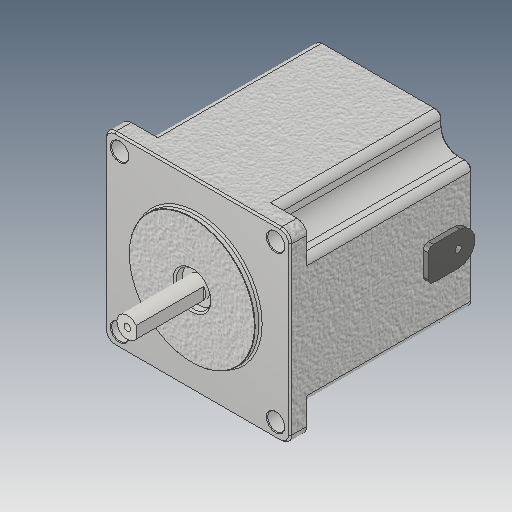
# Autodesk Inventor part: 23hs6403
Saved by Autodesk Inventor 2019 (Build 230136000, 136)
## iProperties
Created: 2018-10-14
Part Number: 23hs6403
Material: Generic
Document SubType Name: Modeling
Designer: LillaHunden
Density: 1 g/cm^3
Appearance: Default
Mass: 158.611 g
Surface Area: 187.385 cm^2
Volume: 158.611 cm^3
Author: LillaHunden
Autodesk Inventor part; units mm, degrees
ref_plane "YZ Plane" through (0, 0, 0) normal (1, 0, 0) x (0, 1, 0)
ref_plane "XZ Plane" through (0, 0, 0) normal (0, 1, 0) x (-1, 0, 0)
ref_plane "XY Plane" through (0, 0, 0) normal (0, 0, 1) x (1, 0, 0)
sketch "Sketch1" plane through (0, 0, 0) normal (0, 0, 1) x (1, 0, 0)
  line L0 (-28, -28) -> (28, -28)
  line L1 (28, -28) -> (28, 28)
  line L2 (28, 28) -> (-28, 28)
  line L3 (-28, 28) -> (-28, -28)
  line L4 (-28, -28) -> (28, 28) construction
  line L5 (28, -28) -> (-28, 28) construction
  point P0 (0, 0)
  dimension "d0" = 56
  dimension "d1" = 56
  constraints: 12 end point, 2 midpoint, 2 parallel, 1 horizontal, 1 perpendicular
  measures "d0" distance of L2.end L1.end
  measures "d1" distance of L1.end L0.end
extrude "Extrusion1" add sketch "Sketch1" along normal blind 55
sketch "Sketch2" plane through (0, 0, 55) normal (0, 0, 1) x (1, 0, 0)
  circle A0 centre (0, 0) radius 19
  dimension "d4" = 38
  constraints: 1 centre point, 1 coincident
  measures "d4" diameter of A0
extrude "Extrusion2" add sketch "Sketch2" along normal blind 1.7
fillet "Fillet1" radius 0.5 1 edges at (-19, 0, 55)
fillet "Fillet2" radius 0.1 1 edges at (-19, 0, 56.7)
sketch "Sketch3" plane through (0, 0, 56.7) normal (0, 0, 1) x (1, 0, 0)
  circle A0 centre (0, 0) radius 3.18
  dimension "d9" = 6.36
  constraints: 1 centre point, 1 coincident
  measures "d9" diameter of A0
extrude "Extrusion3" add sketch "Sketch3" along normal blind 19.5
sketch "Sketch4" plane through (0, 0, 56.7) normal (0, 0, 1) x (1, 0, 0)
  circle A0 centre (0, 0) radius 3.18 projected
  circle A1 centre (0, 0) radius 5.25
  dimension "d12" = 10.5
  constraints: 1 centre point, 1 coincident
  measures "d12" diameter of A1
extrude "Extrusion4" cut sketch "Sketch4" against normal blind 2.4
chamfer "Chamfer1" distance 0.5 angle 45 1 edges at (-5.25, 0, 56.7)
sketch "Sketch5" plane through (0, 0, 76.2) normal (0, 0, 1) x (1, 0, 0)
  circle A0 centre (0, 0) radius 1
  dimension "d18" = 2
  constraints: 1 centre point, 1 coincident
  measures "d18" diameter of A0
extrude "Extrusion5" cut sketch "Sketch5" against normal blind 2.4
draft "FaceDraft1" angle -20 pull direction (0, 0, -1) faces at (0.9871, -0.1604, 74.6) fixed edges at (-1, 0, 76.2)
sketch "Sketch6" plane through (0, 0, 55) normal (0, 0, 1) x (1, 0, 0)
  line L0 (-23.57, -23.57) -> (23.57, -23.57) construction
  line L1 (23.57, -23.57) -> (23.57, 23.57) construction
  line L2 (23.57, 23.57) -> (-23.57, 23.57) construction
  line L3 (-23.57, 23.57) -> (-23.57, -23.57) construction
  circle A0 centre (0, 0) radius 1 construction
  line L4 (-23.57, -23.57) -> (23.57, 23.57) construction
  line L5 (23.57, -23.57) -> (-23.57, 23.57) construction
  circle A1 centre (-23.57, 23.57) radius 2.6
  circle A2 centre (23.57, 23.57) radius 2.6
  circle A3 centre (23.57, -23.57) radius 2.6
  circle A4 centre (-23.57, -23.57) radius 2.6
  dimension "d22" = 47.14
  dimension "d23" = 47.14
  dimension "d24" = 5.2
  dimension "d25" = 5.2
  dimension "d26" = 5.2
  dimension "d27" = 5.2
  constraints: 12 end point, 4 centre point, 4 coincident, 2 midpoint, 2 parallel, 1 horizontal, 1 perpendicular
  measures "d22" distance of L2.end L1.end
  measures "d23" distance of L1.end L0.end
  measures "d24" diameter of A1
  measures "d25" diameter of A4
  measures "d26" diameter of A3
  measures "d27" diameter of A2
extrude "Extrusion6" cut sketch "Sketch6" against normal through all
chamfer "Chamfer2" distance 0.2 angle 45 4 edges at (-26.17, 23.57, 55) (20.97, 23.57, 55) (20.97, -23.57, 55) (-26.17, -23.57, 55)
sketch "Sketch7" plane through (0, 0, 0) normal (0, 0, -1) x (-1, 0, 0)
  circle A0 centre (0, 0) radius 1 projected
  circle A1 centre (0, 0) radius 5.2
  dimension "d33" = 10.4
  constraints: 1 centre point, 1 coincident
  measures "d33" diameter of A1
extrude "Extrusion7" cut sketch "Sketch7" against normal blind 5.3 contours A0 | A1
fillet "Fillet3" radius 3 4 edges at (-28, -28, 27.5) (-28, 28, 27.5) (28, 28, 27.5) (28, -28, 27.5)
sketch "Sketch8" plane through (0, 0, 0) normal (0, 0, -1) x (-1, 0, 0)
  arc A0 (-28, -25) -> (-25, -28) centre (-25, -25) ccw construction
  line L0 (25, -28) -> (-25, -28) construction
  arc A1 (25, -28) -> (28, -25) centre (25, -25) ccw construction
  line L1 (28, 25) -> (28, -25) construction
  arc A2 (28, 25) -> (25, 28) centre (25, 25) ccw construction
  line L2 (-25, 28) -> (25, 28) construction
  arc A3 (-25, 28) -> (-28, 25) centre (-25, 25) ccw construction
  line L3 (-28, -25) -> (-28, 25) construction
  circle A4 centre (0, 0) radius 5.2 construction
  circle A5 centre (-23.57, -23.57) radius 2.6 construction
  circle A6 centre (23.57, 23.57) radius 2.6 construction
  circle A7 centre (-23.57, 23.57) radius 2.6 construction
  circle A8 centre (23.57, -23.57) radius 2.6 construction
  line L4 (19, -19) -> (-19, -19) construction
  line L5 (-19, -19) -> (-19, 19) construction
  line L6 (-19, 19) -> (19, 19) construction
  line L7 (19, 19) -> (19, -19) construction
  circle A9 centre (0, 0) radius 0.1265 construction
  line L8 (19, -19) -> (-19, 19) construction
  line L9 (-19, -19) -> (19, 19) construction
  line L10 (19, -19) -> (19, -28)
  line L11 (25, -28) -> (-25, -28) projected
  line L12 (-19, -19) -> (-19, -28)
  line L13 (-19, -19) -> (-28, -19)
  line L14 (-19, 19) -> (-28, 19)
  line L15 (-28, -25) -> (-28, 25) projected
  line L16 (-19, 19) -> (-19, 28)
  line L17 (19, 19) -> (19, 28)
  line L18 (-25, 28) -> (25, 28) projected
  line L19 (19, 19) -> (28, 19)
  line L20 (19, -19) -> (28, -19)
  line L21 (28, 25) -> (28, -25) projected
  arc A10 (25, -28) -> (28, -25) centre (25, -25) ccw projected
  arc A11 (28, 25) -> (25, 28) centre (25, 25) ccw projected
  arc A12 (-25, 28) -> (-28, 25) centre (-25, 25) ccw projected
  arc A13 (-28, -25) -> (-25, -28) centre (-25, -25) ccw projected
  dimension "d37" = 38
  dimension "d38" = 38
  constraints: 28 end point, 13 point on line, 3 parallel, 3 perpendicular, 2 midpoint, 1 horizontal
  measures "d37" distance of L5.end L6.end
  measures "d38" distance of L4.end L5.end
extrude "Extrusion8" cut sketch "Sketch8" against normal blind 50 contours L19 L17 L18 A11 L21
fillet "Fillet4" radius 5 1 edges at (-19, 19, 25)
fillet "Fillet5" radius 2 2 edges at (-19, 28, 25) (-28, 19, 25)
pattern_circular "Circular Pattern1" count 4 over 360 about axis through (0, 0, 0) along (0, 0, 1) of "Extrusion8"
fillet "Fillet6" radius 2 6 edges at (19, 28, 25) (28, 19, 25) (28, -19, 25) (19, -28, 25) (-28, -19, 25) (-19, -28, 25)
fillet "Fillet7" radius 5 3 edges at (-19, -19, 25) (19, -19, 25) (19, 19, 25)
sketch "Sketch9" plane through (28, -25, 55) normal (1, 0, 0) x (0, 0, -1)
  circle A0 centre (49.2162, 25) radius 5
  line L0 (40.2162, 20) -> (49.7, 20)
  line L1 (49.7, 20) -> (49.7, 30)
  line L2 (49.7, 30) -> (40.2162, 30)
  line L3 (40.2162, 30) -> (40.2162, 20)
  line L4 (55, 8) -> (55, 42) projected
  point P0 (55, 25)
  point P1 (55, 25)
  dimension "d48" = 10
  dimension "d49" = 9
  constraints: 8 end point, 2 parallel, 2 tangent, 1 centre point, 1 horizontal, 1 horizontal alignment, 1 midpoint, 1 perpendicular
  measures "d48" diameter of A0
  measures "d49" distance from line of L3 A0.centre
extrude "Extrusion9" add sketch "Sketch9" along normal blind 1.5
fillet "Fillet8" radius 1.5 2 edges at (28.75, 5, 14.7838) (28.75, -5, 14.7838)
sketch "Sketch10" plane through (29.5, -25, 55) normal (1, 0, 0) x (0, 0, -1)
  circle A0 centre (49.2162, 25) radius 1
  arc A1 (49.7, 20.0235) -> (49.7, 29.9765) centre (49.2162, 25) ccw projected
  point P0 (55, 25)
  dimension "d53" = 2
  constraints: 1 centre point, 1 concentric
  measures "d53" diameter of A0
extrude "Extrusion10" cut sketch "Sketch10" against normal blind 3
sketch "Sketch11" plane through (0, 0, 76.2) normal (0, 0, 1) x (1, 0, 0)
  circle A0 centre (0, 0) radius 3.18 projected
  line L0 (2.62, 1.8022) -> (2.62, -1.8022)
  dimension "d56" = 5.8
  constraints: 2 end point, 2 point on circle, 1 vertical
extrude "Extrusion11" cut sketch "Sketch11" against normal blind 20.5 contours A0 L0 picked at (2.7223, -0.4144)
chamfer "Chamfer3" distance 0.5 angle 45 8 edges at (-28, 0, 55) (-27.1213, -27.1213, 55) (0, -28, 55) (27.1213, -27.1213, 55) (28, 0, 55) (27.1213, 27.1213, 55) (0, 28, 55) (-27.1213, 27.1213, 55)
chamfer "Chamfer4" distance 0.5 angle 45 24 edges at (0, 28, 0) (-18.4142, 27.4142, 0) (-19, 25, 0) (-20.4645, 20.4645, 0) (-25, 19, 0) (-27.4142, 18.4142, 0) (-28, 0, 0) (-27.4142, -18.4142, 0) (-25, -19, 0) (-20.4645, -20.4645, 0) (-19, -25, 0) (-18.4142, -27.4142, 0) (0, -28, 0) (18.4142, -27.4142, 0) (19, -25, 0) (20.4645, -20.4645, 0) (25, -19, 0) (27.4142, -18.4142, 0) (28, 0, 0) (27.4142, 18.4142, 0) (25, 19, 0) (20.4645, 20.4645, 0) (19, 25, 0) (18.4142, 27.4142, 0)
equation "\"d25\" = d24"
equation "\"d26\" = d25"
equation "\"d27\" = d24"
body "Solid1"
